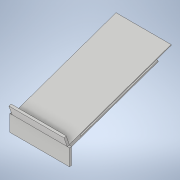
# Autodesk Inventor part: cover
Saved by Autodesk Inventor 2021 (Build 250183000, 183)
## iProperties
Created: 2019-01-15
Part Number: cover
Material: 常规
Document SubType Name: Modeling
Designer: Guo Xin
Density: 1 g/cm^3
Appearance: 默认
Author: Guo Xin
Autodesk Inventor part; units mm, degrees
ref_plane "YZ Plane" through (0, 0, 0) normal (1, 0, 0) x (0, 1, 0)
ref_plane "XZ Plane" through (0, 0, 0) normal (0, 1, 0) x (-1, 0, 0)
ref_plane "XY Plane" through (0, 0, 0) normal (0, 0, 1) x (1, 0, 0)
sketch "草图1" plane through (0, 0, 0) normal (1, 0, 0) x (0, 1, 0)
  line L0 (-7.0511, 44.9164) -> (14.9489, 44.9164)
  line L1 (59.1261, -96.2836) -> (10.702, 41.9164)
  line L2 (10.702, 41.9164) -> (-7.0511, 41.9164)
  line L3 (-7.0511, 41.9164) -> (-7.0511, 44.9164)
  line L4 (57.8575, -77.5428) -> (14.9489, 44.9164)
  line L5 (63.8448, -94.6302) -> (59.1261, -96.2836)
  line L6 (63.8448, -94.6302) -> (57.8575, -77.5428)
  line L7 (10.702, 41.9164) -> (10.702, 44.9164)
  line L8 (14.9489, 44.9164) -> (14.9489, 41.9164)
  point P0 (0, 0)
  dimension "d1" = 3
  dimension "d2" = 109.31
  dimension "d3" = 138.2
  dimension "d10" = 5
  dimension "d90" = 22
  constraints: 18 end point, 3 perpendicular, 2 parallel, 1 horizontal, 1 point on line, 1 vertical
  measures "d1" distance between parallel lines of L2 L0
  measures "d2" angle of L2 L1
  measures "d3" vertical distance of L1.start L1.end
  measures "d10" distance between parallel lines of L1 L4
  measures "d90" distance between parallel lines of L8 L3
extrude "拉伸1" add sketch "草图1" along normal blind 74
sketch "草图4" plane through (0, 14.9489, 44.9164) normal (0, 0.9437433, 0.3306791) x (1, 0, 0)
  line L0 (74, 3) -> (0, 3)
  line L1 (0, 3) -> (0, 0)
  line L2 (0, 0) -> (74, 0)
  line L3 (74, 0) -> (74, 3)
  line L4 (0, 0) -> (74, 0) projected
  line L5 (74, 147.865) -> (74, 0) projected
  line L6 (0, 0) -> (0, 147.865) projected
  point P0 (0, 37.4463)
  point P1 (67.5, 129.877)
  point P2 (0, 129.877)
  dimension "d11" = 3
  constraints: 8 end point, 2 collinear, 2 parallel, 1 horizontal, 1 perpendicular, 1 vertical, 1 other
  measures "d11" distance between parallel lines of L2 L0
extrude "拉伸3" add sketch "草图4" along normal blind 13
sketch "草图5" plane through (74, 0, 0) normal (1, 0, 0) x (0, 0, -1)
  line L0 (-27.5984, 19.9574) -> (113.9631, 69.5592)
  line L1 (113.9631, 69.5592) -> (114.7237, 67.3886)
  line L2 (114.7237, 67.3886) -> (-26.8378, 17.7868)
  line L3 (-26.8378, 17.7868) -> (-27.5984, 19.9574)
  line L4 (94.6302, 63.8448) -> (-42.0852, 15.9409) projected
  line L5 (-42.0852, 15.9409) -> (-40.3206, 10.9047)
  point P0 (0, 0)
  point P1 (78.0607, 56.3152)
  dimension "d15" = 1
  dimension "d16" = 150
  dimension "d17" = 2.3
  dimension "d22" = 15
  constraints: 10 end point, 2 parallel, 2 perpendicular, 2 other
  measures "d16" distance between parallel lines of L1 L3
  measures "d17" distance between parallel lines of L2 L0
  measures "d22" distance between parallel lines of L5 L3
extrude "拉伸4" cut sketch "草图5" against normal blind 5
sketch "草图6" plane through (0, 0, 0) normal (-1, 0, 0) x (0, 0, 1)
  line L0 (-113.9631, 69.5592) -> (27.5984, 19.9574)
  line L1 (27.5984, 19.9574) -> (26.8378, 17.7868)
  line L2 (26.8378, 17.7868) -> (-114.7237, 67.3886)
  line L3 (-114.7237, 67.3886) -> (-113.9631, 69.5592)
  line L4 (42.0852, 15.9409) -> (-94.6302, 63.8448) projected
  line L5 (42.0852, 15.9409) -> (38.373, 5.3464)
  point P0 (0, 0)
  point P1 (-78.0607, 56.3152)
  dimension "d20" = 1
  dimension "d21" = 2.3
  dimension "d23" = 15
  dimension "d24" = 150
  constraints: 10 end point, 3 perpendicular, 2 other
  measures "d21" distance between parallel lines of L2 L0
  measures "d23" distance between parallel lines of L5 L1
  measures "d24" distance between parallel lines of L1 L3
extrude "拉伸5" cut sketch "草图6" against normal blind 5
sketch "草图8" plane through (74, 0, 0) normal (1, 0, 0) x (0, 0, -1)
  line L0 (96.2836, 59.1261) -> (95.7214, 60.7304)
  line L1 (95.7214, 60.7304) -> (76.8465, 54.1168)
  line L2 (76.8465, 54.1168) -> (77.4087, 52.5125)
  line L3 (77.4087, 52.5125) -> (96.2836, 59.1261)
  line L4 (96.2836, 59.1261) -> (95.7214, 60.7304) projected
  line L5 (-41.9164, 10.702) -> (96.2836, 59.1261) projected
  line L6 (95.7214, 60.7304) -> (-26.8378, 17.7868) projected
  point P0 (0, 0)
  point P1 (84.6027, 53.1652)
  dimension "d32" = 20
  constraints: 8 end point, 2 collinear, 2 parallel, 1 perpendicular, 2 other
  measures "d32" distance between parallel lines of L0 L2
extrude "拉伸7" cut sketch "草图8" against normal blind 100
sketch "草图9" plane through (0, -7.0511, 44.9164) normal (0, 0, 1) x (1, 0, 0)
  line L0 (-3, 22) -> (77, 22)
  line L1 (77, 22) -> (77, 0)
  line L2 (77, 0) -> (-3, 0)
  line L3 (-3, 0) -> (-3, 22)
  line L4 (0, 22) -> (74, 22) projected
  line L5 (0, 0) -> (74, 0) projected
  line L6 (0, 0) -> (0, 22) projected
  line L7 (74, 22) -> (74, 0) projected
  point P0 (0, 7.0511)
  dimension "d35" = 3
  dimension "d36" = 3
  constraints: 8 end point, 2 collinear, 2 parallel, 1 horizontal, 1 perpendicular
  measures "d35" distance between parallel lines of L6 L3
  measures "d36" distance between parallel lines of L7 L1
extrude "拉伸8" add sketch "草图9" against normal blind 3 contours L0 L6 L2 L3 | L0 L1 L2 L7
sketch "草图10" plane through (74, 10.702, 41.9164) normal (0, 0, -1) x (-1, 0, 0)
  line L0 (10, -16.2531) -> (64, -16.2531)
  line L1 (64, -16.2531) -> (64, -17.7531)
  line L2 (64, -17.7531) -> (10, -17.7531)
  line L3 (10, -17.7531) -> (10, -16.2531)
  line L4 (-3, -17.7531) -> (77, -17.7531) projected
  line L5 (0, 0) -> (0, 41.8104) projected
  line L6 (77, -17.7531) -> (77, 4.2469) projected
  line L7 (74, 41.8104) -> (74, 0) projected
  point P0 (74, -10.702)
  point P1 (0, 38.8623)
  point P2 (67.5, 38.8623)
  point P3 (80, 48.424)
  dimension "d39" = 1.5
  dimension "d40" = 10
  dimension "d55" = 10
  constraints: 8 end point, 2 parallel, 1 collinear, 1 horizontal, 1 perpendicular, 1 other
  measures "d39" distance between parallel lines of L2 L0
  measures "d40" distance between parallel lines of L5 L3
extrude "拉伸9" add sketch "草图10" along normal blind 10
sketch "草图11" plane through (-3, -7.0511, 44.9164) normal (0, -1, 0) x (1, 0, 0)
  line L0 (77, -3) -> (77, -122.3251) projected
  line L1 (3, -122.3251) -> (3, -3) projected
  line L2 (0, 0) -> (80, 0) projected
  line L3 (80, -3) -> (67, -3) projected
  line L4 (13, -3) -> (13, -13) projected
  line L5 (67, -13) -> (13, -13) projected
  point P0 (3, -44.9164)
  point P1 (59, -7)
  point P2 (21, -7)
  point P3 (70.75, -123.9692)
  point P4 (3.25, -123.9692)
  point P5 (3.25, -141.2)
  dimension "d44" = 18
  dimension "d45" = 18
  dimension "d53" = 7
  dimension "d54" = 7
  dimension "d56" = 3
  dimension "d57" = 8
  dimension "d58" = 6
  constraints: 2 other
  measures "d53" distance from line of L2 point (59, -7)
  measures "d54" distance from line of L2 point (21, -7)
  measures "d56" distance between parallel lines of L2 L3
  measures "d57" distance from line of L4 point (21, -7)
  measures "d58" distance from line of L5 point (21, -7)
hole "孔1" at (56, -7.0511, 37.9164) at (18, -7.0511, 37.9164) direction (0, 1, 0) diameter 2.013 depth 2 tip angle 118 thread size "M2.5x0.45" class "6H" standard "ANSI Metric M Profile"
sketch "草图21" plane through (74, 0, 0) normal (1, 0, 0) x (0, 0, -1)
  line L0 (-42.0852, 15.9409) -> (94.6302, 63.8448) projected
  line L1 (94.6302, 63.8448) -> (95.8266, 63.8448)
  line L2 (95.8266, 63.8448) -> (95.8266, 58.5781)
  line L3 (95.8266, 58.5781) -> (94.6302, 58.5781)
  line L4 (94.6302, 58.5781) -> (94.6302, 63.8448)
  point P0 (0, 0)
  constraints: 8 end point, 2 parallel, 1 horizontal, 1 perpendicular
extrude "拉伸14" cut sketch "草图21" against normal blind 150
sketch "草图22" plane through (0, 10.702, 41.9164) normal (0, -0.9437433, -0.3306791) x (1, 0, 0)
  line L0 (5, -145.2818) -> (69, -145.2818) projected
  line L1 (64, -10.7184) -> (10, -10.7184)
  line L2 (10, -10.7184) -> (10, -145.2818)
  line L3 (10, -145.2818) -> (64, -145.2818)
  line L4 (64, -145.2818) -> (64, -10.7184)
  line L5 (74, 0) -> (74, -126.4381) projected
  line L6 (0, -126.4381) -> (0, 0) projected
  line L7 (74, -16.5731) -> (74, -146.0877) projected
  line L8 (69, -145.2818) -> (69, -146.0877) projected
  point P0 (0, -36.0194)
  point P1 (67.5, -127.0584)
  point P2 (0, -127.0584)
  point P3 (74, -146.0877)
  point P4 (64, -145.2818)
  point P5 (80, -133.0485)
  point P6 (0, -133.0485)
  point P7 (12, -145.2818)
  point P8 (0, -146.4381)
  point P9 (64, -145.2818)
  dimension "d74" = 10
  dimension "d75" = 10
  dimension "d76" = 5
  constraints: 8 end point, 2 parallel, 1 horizontal, 1 perpendicular, 1 point on line, 2 other
  measures "d75" distance between parallel lines of L6 L2
extrude "拉伸15" cut sketch "草图22" against normal blind 2.5
sketch "草图25" plane through (0, 10.702, 41.9164) normal (0, -0.9437433, -0.3306791) x (1, 0, 0)
  line L0 (0, -126.4381) -> (0, 0) projected
  line L1 (69.9045, -127.7568) -> (0, -127.7568)
  line L2 (0, -127.7568) -> (0, -133.0485)
  line L3 (0, -133.0485) -> (69.9045, -133.0485)
  line L4 (69.9045, -133.0485) -> (69.9045, -127.7568)
  point P0 (0, -36.0194)
  point P1 (0, -127.7568)
  constraints: 8 end point, 2 parallel, 1 horizontal, 1 perpendicular
extrude "拉伸16" cut sketch "草图25" against normal blind 1.7
